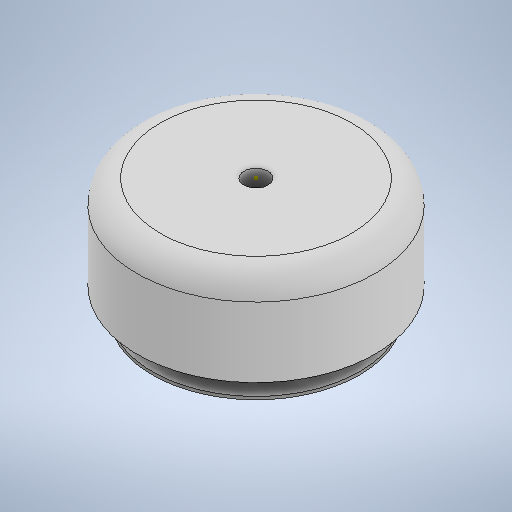
# Autodesk Inventor part: Water_Sensor_Cap
Saved by Autodesk Inventor 2025 (Build 290162000, 162)
## iProperties
Created: 2024-06-19
Part Number: Water_Sensor_Cap
Material: Generic
Document SubType Name: Modeling
Designer: track
Density: 1 g/cm^3
Appearance: Default
Mass: 56.6087 g
Surface Area: 245.5 cm^2
Volume: 56.6087 cm^3
Author: track
## iProperties of the stored document Water_Sensor_Cap_3DPrint.ipt
Created: 2024-06-19
Part Number: Water_Sensor_Cap_3DPrint
Material: Generic
Document SubType Name: Modeling
Designer: track
Density: 1 g/cm^3
Appearance: Default
Author: track
Autodesk Inventor part; units mm, degrees
ref_plane "YZ Plane" through (0, 0, 0) normal (1, 0, 0) x (0, 1, 0)
ref_plane "XZ Plane" through (0, 0, 0) normal (0, 1, 0) x (-1, 0, 0)
ref_plane "XY Plane" through (0, 0, 0) normal (0, 0, 1) x (1, 0, 0)
sketch "Sketch1" plane through (0, 0, 0) normal (0, 1, 0) x (-1, 0, 0)
  circle A0 centre (0, 0) radius 30.48
  circle A1 centre (0, 0) radius 32.48
  dimension "d0" = 60.96
  dimension "d2" = 2
  constraints: 2 centre point, 2 coincident
  measures "d0" diameter of A0
  measures "d2" radial gap between concentric circles of A1 A0
extrude "Extrusion1" add sketch "Sketch1" along normal blind 19.05
sketch "Sketch2" plane through (0, 19.05, 0) normal (0, 1, 0) x (1, 0, 0)
  circle A0 centre (0, 0) radius 32.48
  circle A1 centre (0, 0) radius 32.48 projected
  constraints: 1 centre point, 1 coincident, 1 concentric
extrude "Extrusion2" add sketch "Sketch2" along normal blind 6.35
fillet "Fillet1" radius 6.35 1 edges at (-32.48, 25.4, 0)
sketch "Sketch3" plane through (0, 25.4, 0) normal (0, 1, 0) x (1, 0, 0)
  point P0 (0, 0)
sketch "Sketch6" plane through (0, 25.4, 0) normal (0, 1, 0) x (1, 0, 0)
  circle A0 centre (0, 0) radius 3.302
  dimension "d15" = 6.604
  constraints: 1 centre point, 1 coincident
  measures "d15" diameter of A0
extrude "Extrusion5" cut sketch "Sketch6" against normal up to surface (6.35 mm away)
sketch "Sketch9" plane through (0, 19.05, 0) normal (0, -1, 0) x (1, 0, 0)
  point P0 (0, 0)
sketch "Sketch10" plane through (0, 0, 0) normal (0, 0, 1) x (1, 0, 0)
  line L0 (-30.48, 19.05) -> (30.48, 19.05) projected
  line L1 (-20.66, 19.05) -> (-20.66, -11.43)
  line L2 (-20.66, -11.43) -> (-28.28, -11.43)
  line L3 (-28.28, -11.43) -> (-28.28, 19.05)
  line L4 (-20.66, 19.05) -> (-28.28, 19.05)
  line L5 (-26.13, 25.4) -> (26.13, 25.4) projected
  line L6 (0, 25.4) -> (0, 0)
  line L7 (32.48, 0) -> (-32.48, 0) projected
  line L8 (-30.48, 0) -> (-30.48, 19.05)
  line L9 (-20.66, -11.43) -> (-28.28, -7.0306)
  dimension "d29" = 7.62
  dimension "d31" = 2.2
  dimension "d32" = 30.48
  dimension "d33" = 30
  constraints: 14 end point, 4 perpendicular, 4 point on line, 2 vertical, 1 midpoint
  measures "d29" distance between parallel lines of L1 L3
  measures "d31" distance between parallel lines of L3 L8
  measures "d32" distance of L2.end L3.end
  measures "d33" angle of L2 L9
revolve "Revolution2" add sketch "Sketch10" angle 360 about axis through (0, 25.4, 0) along (0, -1, 0) contours L0 L1 L7 L3 | L7 L1 L9 L3
sketch "Sketch11" plane through (0, 0, 0) normal (0, 0, 1) x (1, 0, 0)
  line L0 (28.28, 19.05) -> (28.28, -7.0306) projected
  line L1 (28.28, -7.0306) -> (28.28, 25.4)
  circle A0 centre (28.272, -3.8556) radius 2.3813
  circle A1 centre (28.272, 2.4944) radius 2.3813
  line L2 (-28.28, -7.0306) -> (28.28, -7.0306) projected
  line L3 (-20.66, -11.43) -> (20.66, -11.43) projected
  line L4 (0, -11.43) -> (0, 25.4)
  line L5 (-26.13, 25.4) -> (26.13, 25.4) projected
  line L6 (28.272, 2.4944) -> (28.272, -3.8556)
  line L7 (30.48, 19.05) -> (30.48, 0) projected
  line L8 (29.972, 0) -> (29.972, 19.05)
  line L9 (29.972, 19.05) -> (29.972, 0) projected
  point P0 (0, 0)
  point P1 (28.28, -1.4744)
  point P2 (28.28, 0.1132)
  point P3 (27.772, -0.6806)
  point P4 (28.28, 4.8756)
  point P5 (28.28, -6.2368)
  dimension "d35" = 3.175
  dimension "d36" = 6.35
  dimension "d37" = 4.7625
  dimension "d38" = 4.7625
  dimension "d41" = 1.7
  constraints: 8 end point, 2 centre point, 2 midpoint, 1 parallel, 1 point on line, 1 vertical, 4 other
  measures "d35" distance from line of L2 L6.end
  measures "d36" distance of L6.end L6.start
  measures "d37" diameter of A1
  measures "d38" diameter of A0
  measures "d41" distance between parallel lines of L6 L8
revolve "Revolution3" cut sketch "Sketch11" angle 360 about axis through (0, -11.43, 0) along (0, 1, 0) picked at (27.4892, -3.7611) contours L0 A1 | L0 A0
body "Solid1"
